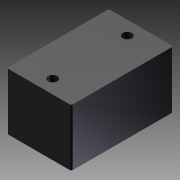
# Autodesk Inventor part: S114-body
Saved by Autodesk Inventor 2011 SP1 (Build 150282100, 282)
## iProperties
Created: 2013-12-24
Part Number: S114-body
Catalog Web Link: www.cadenas.de
Description: S Low Series body-Low Capacity Standard Size Toggles -body
Vendor: NKKSWITCHES
Document SubType Name: Modeling
Designer: PARTuser1
Manufacturer: NKKSWITCHES
Density: 1 g/cm^3
Category: PARTsolutions
Company: NKKSWITCHES
Title: S114-body
Author: Cadenas PARTsolutions
Comments: Low Capacity Standard Size Toggles -body
PSOL_IDENT_0: {$CADENAS_DATA\23d-libs\nkkswitches\toggle\s\parts\s_low_body.prj},171 {VTYP=3D},{NB=S114-body},{LIN
PSOL_IDENT_1: A=S114-body},{NN=S Low Series body},{DATE=05.04.2013 11:25:07},{GEOMDATE=05.04.2013 13:23:00},{VERSI
PSOL_IDENT_2: ON=},{LINEID=10},{LINESUBID=-1},{WBVAR=}  {NB=S114-body},{LINA=S114-body},{KT=DUMMY},{PN=S114},{MDL=
PSOL_IDENT_3: S114}
CNS_NN: S Low Series body
CNS_NT: Low Capacity Standard Size Toggles -body
CNS_NB: S114-body
CNS_NBSYN: $PN.-body
CNS_LINA: S114-body
CNS_PN: S114
CNS_MDL: S114
SUPPLIER: NKKSWITCHES
ARTICLENO: S114-body
BOMINFO: S114-body
CREATOR: CADENAS GmbH
Autodesk Inventor part; units mm, degrees
sketch "Sketch_1" plane through (0, 0, 0) normal (0, 1, 0) x (-1, 0, 0)
  line L0 (8.8011, -13.3858) -> (8.8011, 13.3858)
  arc A0 (8.8011, 13.3858) -> (8.2931, 13.8938) centre (8.2931, 13.3858) ccw
  line L1 (8.2931, 13.8938) -> (-8.2931, 13.8938)
  arc A1 (-8.2931, 13.8938) -> (-8.8011, 13.3858) centre (-8.2931, 13.3858) ccw
  line L2 (-8.8011, 13.3858) -> (-8.8011, -13.3858)
  arc A2 (-8.8011, -13.3858) -> (-8.2931, -13.8938) centre (-8.2931, -13.3858) ccw
  line L3 (-8.2931, -13.8938) -> (8.2931, -13.8938)
  arc A3 (8.2931, -13.8938) -> (8.8011, -13.3858) centre (8.2931, -13.3858) ccw
  constraints: 8 end point, 8 point on circle, 4 centre point
extrude "Extrusion1" add sketch "Sketch_1" against normal blind 15.494
sketch "Sketch_2" plane through (0, -15.494, 0) normal (0, 1, 0) x (1, 0, 0)
  arc A0 (-4.953, -12.446) -> (-4.699, -12.7) centre (-4.699, -12.446) ccw
  line L0 (-4.699, -12.7) -> (-4.318, -12.7)
  line L1 (-4.318, -12.7) -> (-4.318, -8.89)
  line L2 (-4.318, -8.89) -> (-4.699, -8.89)
  arc A1 (-4.699, -8.89) -> (-4.953, -9.144) centre (-4.699, -9.144) ccw
  line L3 (-4.953, -9.144) -> (-4.953, -12.446)
  constraints: 8 end point, 4 point on circle, 2 centre point
extrude "Extrusion2" cut sketch "Sketch_2" along normal blind 0.254
sketch "Sketch_3" plane through (0, -15.494, 0) normal (0, 1, 0) x (1, 0, 0)
  line L0 (4.318, -12.7) -> (4.699, -12.7)
  arc A0 (4.699, -12.7) -> (4.953, -12.446) centre (4.699, -12.446) ccw
  line L1 (4.953, -12.446) -> (4.953, -9.144)
  arc A1 (4.953, -9.144) -> (4.699, -8.89) centre (4.699, -9.144) ccw
  line L2 (4.699, -8.89) -> (4.318, -8.89)
  line L3 (4.318, -8.89) -> (4.318, -12.7)
  constraints: 8 end point, 4 point on circle, 2 centre point
extrude "Extrusion3" cut sketch "Sketch_3" along normal blind 0.254
sketch "Sketch_4" plane through (0, -15.494, 0) normal (0, 1, 0) x (1, 0, 0)
  line L0 (-4.953, 12.446) -> (-4.953, 9.144)
  arc A0 (-4.953, 9.144) -> (-4.699, 8.89) centre (-4.699, 9.144) ccw
  line L1 (-4.699, 8.89) -> (-4.318, 8.89)
  line L2 (-4.318, 8.89) -> (-4.318, 12.7)
  line L3 (-4.318, 12.7) -> (-4.699, 12.7)
  arc A1 (-4.699, 12.7) -> (-4.953, 12.446) centre (-4.699, 12.446) ccw
  constraints: 8 end point, 4 point on circle, 2 centre point
extrude "Extrusion4" cut sketch "Sketch_4" along normal blind 0.254
sketch "Sketch_5" plane through (0, -15.494, 0) normal (0, 1, 0) x (1, 0, 0)
  line L0 (4.318, 12.7) -> (4.318, 8.89)
  line L1 (4.318, 8.89) -> (4.699, 8.89)
  arc A0 (4.699, 8.89) -> (4.953, 9.144) centre (4.699, 9.144) ccw
  line L2 (4.953, 9.144) -> (4.953, 12.446)
  arc A1 (4.953, 12.446) -> (4.699, 12.7) centre (4.699, 12.446) ccw
  line L3 (4.699, 12.7) -> (4.318, 12.7)
  constraints: 8 end point, 4 point on circle, 2 centre point
extrude "Extrusion5" cut sketch "Sketch_5" along normal blind 0.254
sketch "Sketch6" plane through (0, -15.494, 0) normal (0, -1, 0) x (1, 0, 0)
  point P0 (0, 10.16)
hole "Drilling 1" at (0, -15.494, 10.16) direction (0, 1, 0) diameter 2.5 depth 15.494 counterbore diameter 5.08 counterbore depth 2.032
sketch "Sketch7" plane through (0, -15.494, 0) normal (0, -1, 0) x (1, 0, 0)
  point P0 (0, -10.16)
hole "Drilling 2" at (0, -15.494, -10.16) direction (0, 1, 0) diameter 2.5 depth 15.494 counterbore diameter 5.08 counterbore depth 2.032
ref_plane "screw_m25_2_XY" through (0, -13.462, -10.16) normal (0, 1, 0) x (1, 0, 0)
ref_plane "screw_m25_2_YZ" through (0, -13.462, -10.16) normal (1, 0, 0) x (0, 0, -1)
ref_plane "screw_m25_2_ZX" through (0, -13.462, -10.16) normal (0, 0, -1) x (0, 1, 0)
ref_plane "sscrew_m25_1_XY" through (0, -13.462, 10.16) normal (0, 1, 0) x (1, 0, 0)
ref_plane "sscrew_m25_1_YZ" through (0, -13.462, 10.16) normal (1, 0, 0) x (0, 0, -1)
ref_plane "sscrew_m25_1_ZX" through (0, -13.462, 10.16) normal (0, 0, -1) x (0, 1, 0)
ref_plane "to_dummy_XY" through (0, 0, 0) normal (0, -1, 0) x (1, 0, 0)
ref_plane "to_dummy_YZ" through (0, 0, 0) normal (1, 0, 0) x (0, 0, 1)
ref_plane "to_dummy_ZX" through (0, 0, 0) normal (0, 0, 1) x (0, -1, 0)
ref_plane "to_electric_XY" through (0, -15.24, 0) normal (0, 1, 0) x (1, 0, 0)
ref_plane "to_electric_YZ" through (0, -15.24, 0) normal (1, 0, 0) x (0, 0, -1)
ref_plane "to_electric_ZX" through (0, -15.24, 0) normal (0, 0, -1) x (0, 1, 0)
ref_plane "to_panel_XY" through (0, 0, 0) normal (0, -1, 0) x (1, 0, 0)
ref_plane "to_panel_YZ" through (0, 0, 0) normal (1, 0, 0) x (0, 0, 1)
ref_plane "to_panel_ZX" through (0, 0, 0) normal (0, 0, 1) x (0, -1, 0)
body "Solid1"
